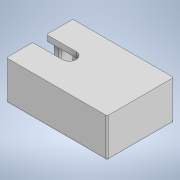
# Autodesk Inventor part: 麥克風蓋
Saved by Autodesk Inventor 2021 (Build 250183000, 183)
## iProperties
Created: 2023-03-09
Part Number: 麥克風蓋
Material: 一般
Document SubType Name: Modeling
Designer: brian
Density: 1 g/cm^3
Appearance: 預設
Author: brian
Autodesk Inventor part; units mm, degrees
ref_plane "YZ Plane" through (0, 0, 0) normal (1, 0, 0) x (0, 1, 0)
ref_plane "XZ Plane" through (0, 0, 0) normal (0, 1, 0) x (-1, 0, 0)
ref_plane "XY Plane" through (0, 0, 0) normal (0, 0, 1) x (1, 0, 0)
sketch "草圖1" plane through (0, 0, 0) normal (0, 1, 0) x (-1, 0, 0)
  line L0 (-76.5, 50.5) -> (76.5, 50.5)
  line L1 (76.5, 50.5) -> (76.5, -50.5)
  line L2 (76.5, -50.5) -> (-76.5, -50.5)
  line L3 (-76.5, -50.5) -> (-76.5, 50.5)
  line L4 (-76.5, 50.5) -> (76.5, -50.5) construction
  line L5 (76.5, 50.5) -> (-76.5, -50.5) construction
  circle A0 centre (31.5, 0) radius 10.5
  line L6 (31.5, 10.5) -> (76.5, 10.5)
  line L7 (31.5, -10.5) -> (76.5, -10.5)
  point P0 (0, 0)
  point P1 (0, 0)
  dimension "d0" = 153
  dimension "d1" = 101
  dimension "d2" = 45
  dimension "d3" = 21
  constraints: 16 end point, 3 midpoint, 3 perpendicular, 2 parallel, 2 point on circle, 2 point on line, 2 tangent, 1 centre point, 1 horizontal, 1 horizontal alignment
  measures "d0" distance of L1.end L2.end
  measures "d1" distance of L0.end L1.end
  measures "d2" distance from line of L1 A0.centre
  measures "d3" diameter of A0
extrude "擠出1" add sketch "草圖1" along normal blind 10 contours L0 L1 L6 A0 L7 L2 L3
sketch "草圖2" plane through (0, 0, 0) normal (0, -1, 0) x (1, 0, 0)
  line L0 (76.5, 50.5) -> (76.5, -50.5) projected
  line L1 (-76.5, 50.5) -> (76.5, 50.5) projected
  line L2 (-76.5, 10.5) -> (-76.5, 50.5) projected
  line L3 (-31.5, 10.5) -> (-76.5, 10.5) projected
  arc A0 (-31.5, -10.5) -> (-31.5, 10.5) centre (-31.5, 0) ccw projected
  line L4 (-76.5, -10.5) -> (-31.5, -10.5) projected
  line L5 (-76.5, -50.5) -> (-76.5, -10.5) projected
  line L6 (76.5, -50.5) -> (-76.5, -50.5) projected
  line L7 (66.5, 40.5) -> (66.5, -40.5)
  line L8 (66.5, -40.5) -> (-66.5, -40.5)
  line L9 (-66.5, -40.5) -> (-66.5, -20.5)
  line L10 (-66.5, -20.5) -> (-31.5, -20.5)
  arc A1 (-31.5, -20.5) -> (-31.5, 20.5) centre (-31.5, 0) ccw
  line L11 (-31.5, 20.5) -> (-66.5, 20.5)
  line L12 (-66.5, 20.5) -> (-66.5, 40.5)
  line L13 (-66.5, 40.5) -> (66.5, 40.5)
  line L14 (-66.5, 20.5) -> (-76.5, 20.5)
  line L15 (-66.5, -20.5) -> (-76.5, -20.5)
  line L16 (-76.5, -50.5) -> (-76.5, -10.5) projected
  point P0 (0, 0)
  dimension "d6" = 10
  constraints: 18 end point, 2 point on circle, 2 point on line, 1 centre point, 1 parallel, 1 perpendicular, 7 other
  measures "d6" distance between parallel lines of L1 L13
extrude "擠出2" add sketch "草圖2" along normal blind 49 contours L0 L6 L5 L15 L9 L8 L7 L13 L12 L14 L2 L1
fillet "圓角1" radius 2 26 edges at (76.5, -19.5, 50.5) (-76.5, -19.5, 50.5) (-76.5, 5, -10.5) (-76.5, 5, 10.5) (-76.5, -19.5, -50.5) (76.5, -19.5, -50.5) (0, -49, 50.5) (0, -49, 40.5) (-76.5, -49, 35.5) (-66.5, -49, 30.5) (-71.5, -49, -20.5) (-71.5, -49, 20.5) (-76.5, -24.5, -20.5) (-66.5, -24.5, -20.5) (-76.5, -49, -35.5) (-66.5, -49, -30.5) (0, -49, -50.5) (0, -49, -40.5) (-76.5, 0, -15.5) (-76.5, 0, 15.5) (-76.5, -24.5, 20.5) (-54, 0, 10.5) (-54, 0, -10.5) (-21, 0, 0) (66.5, -49, 0) (76.5, -49, 0)
